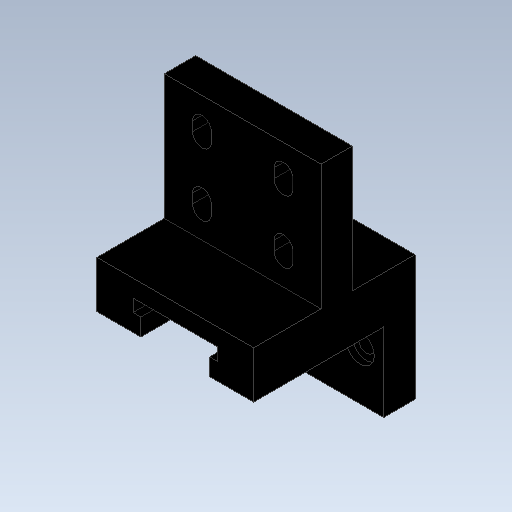
# Autodesk Inventor part: 10-03-029
Saved by Autodesk Inventor 2020 (Build 240168000, 168)
## iProperties
Created: 2019-05-27
Part Number: 10-03-029
Material: Generic
Document SubType Name: Modeling
Designer: Iulian
Density: 1 g/cm^3
Appearance: Default
Description: Suport Intinzator
Mass: 59.2019 g
Surface Area: 181.082 cm^2
Volume: 59.2019 cm^3
Author: Iulian
Subject: 037
Autodesk Inventor part; units mm, degrees
ref_plane "YZ Plane" through (0, 0, 0) normal (1, 0, 0) x (0, 1, 0)
ref_plane "XZ Plane" through (0, 0, 0) normal (0, 1, 0) x (-1, 0, 0)
sketch "Sketch1" plane through (0, 0, 0) normal (1, 0, 0) x (0, 1, 0)
  line L0 (80, 41.5) -> (25, 41.5)
  line L1 (25, 41.5) -> (25, -10)
  line L2 (25, -10) -> (80, -10)
  line L3 (80, -10) -> (80, 41.5)
  line L4 (25, 0) -> (0, 0)
  line L5 (0, 0) -> (0, -10)
  line L6 (0, -10) -> (25, -10)
  line L7 (25, -10) -> (25, 0)
  line L8 (40, 10) -> (80, 10)
  line L9 (80, 10) -> (80, -10)
  line L10 (80, -10) -> (40, -10)
  line L11 (40, -10) -> (40, 10)
  point P0 (25, -10)
  dimension "d0" = 55
  dimension "d1" = 10
  dimension "d3" = 51.5
  dimension "d135" = 25
  dimension "d144" = 20
  dimension "d145" = 40
  constraints: 24 end point, 6 parallel, 3 collinear, 3 horizontal, 3 perpendicular, 1 coincident, 1 point on line
  measures "d0" distance of L0.start L0.end
  measures "d1" distance of L4.end L5.end
  measures "d3" distance of L2.end L0.start
  measures "d135" distance between parallel lines of L1 L5
  measures "d144" distance of L10.end L8.start
  measures "d145" distance of L8.start L8.end
extrude "Extrusion1" add sketch "Sketch1" along normal blind 50 contours L3 L8 L11 L2 L1 L0 | L1 L6 L5 L4
ref_plane "Work Plane1" through (0, 25, 8.75) normal (0, 0, 1) x (1, 0, 0)
sketch "Sketch23" plane through (0, 25, 41.5) normal (0, 0, 1) x (1, 0, 0)
  line L0 (38.5, 9.5) -> (11.5, 9.5)
  line L1 (0, 0) -> (50, 0) projected
  line L2 (38.5, 9.5) -> (38.5, 5.5)
  line L3 (38.5, 5.5) -> (36, 5.5)
  line L4 (36, 5.5) -> (36, 0)
  line L5 (0, 0) -> (50, 0) projected
  line L6 (11.5, 9.5) -> (11.5, 5.5)
  line L7 (11.5, 5.5) -> (14, 5.5)
  line L8 (14, 5.5) -> (14, 0)
  point P0 (0, -25)
  point P1 (25, 9.5)
  point P2 (25, 0)
  point P3 (14, 0)
  point P4 (36, 0)
  dimension "d149" = 9.5
  dimension "d150" = 4
  dimension "d151" = 2.5
  dimension "d152" = 27
  constraints: 14 end point, 3 parallel, 3 perpendicular, 2 equal length, 2 midpoint, 2 point on line, 1 vertical, 1 vertical alignment
  measures "d149" distance between parallel lines of L0 L1
  measures "d150" distance of L0.start L2.end
  measures "d151" distance of L2.end L3.end
  measures "d152" distance of L0.start L0.end
extrude "Extrusion16" cut sketch "Sketch23" against normal up to surface (41.5 mm away)
sketch "Sketch24" plane through (50, 0, 0) normal (1, 0, 0) x (0, 0, -1)
  line L0 (-20, 45) -> (-41.5, 45)
  line L1 (-41.5, 45) -> (-41.5, 80)
  line L2 (-41.5, 80) -> (-20, 80)
  line L3 (-20, 80) -> (-20, 45)
  line L4 (-10, 40) -> (-10, 80) projected
  line L5 (10, 40) -> (-10, 40) projected
  line L6 (-41.5, 80) -> (-41.5, 25) projected
  line L7 (-10, 80) -> (-41.5, 80) projected
  point P0 (0, 0)
  dimension "d155" = 10
  dimension "d156" = 5
  constraints: 8 end point, 2 collinear, 2 parallel, 1 horizontal, 1 perpendicular
  measures "d155" distance between parallel lines of L4 L3
  measures "d156" distance between parallel lines of L0 L5
extrude "Extrusion17" cut sketch "Sketch24" against normal through all
sketch "Sketch25" plane through (0, 0, 0) normal (0, 0, 1) x (1, 0, 0)
  circle A0 centre (7.5, 15.5) radius 2.5
  circle A1 centre (42.5, 15.5) radius 2.5
  line L0 (0, 0) -> (50, 0) projected
  line L1 (50, 25) -> (50, 0) projected
  dimension "d162" = 5
  dimension "d163" = 15.5
  dimension "d164" = 7.5
  dimension "d165" = 35
  constraints: 2 centre point, 1 equal radius, 1 horizontal alignment
  measures "d162" diameter of A1
  measures "d163" distance from line of L0 A1.centre
  measures "d164" distance from line of L1 A1.centre
  measures "d165" distance of A0.centre A1.centre
hole "Hole5" at (7.5, 15.5, 0) at (42.5, 15.5, 0) direction (0, 0, -1) diameter 5 end through all counterbore diameter 9 counterbore depth 2
move faces "Move6" translate (0, -5, 0) faces at (33.3333, 45, 34.3333)
sketch "Sketch26" plane through (0, 80, 20) normal (0, 0, 1) x (1, 0, 0)
  line L0 (38, -31.5) -> (38, -28.5) construction
  line L1 (41, -31.5) -> (41, -28.5)
  line L2 (35, -28.5) -> (35, -31.5)
  arc A0 (35, -31.5) -> (41, -31.5) centre (38, -31.5) ccw
  arc A1 (41, -28.5) -> (35, -28.5) centre (38, -28.5) ccw
  line L3 (12, -31.5) -> (12, -28.5) construction
  line L4 (15, -31.5) -> (15, -28.5)
  line L5 (9, -28.5) -> (9, -31.5)
  arc A2 (9, -31.5) -> (15, -31.5) centre (12, -31.5) ccw
  arc A3 (15, -28.5) -> (9, -28.5) centre (12, -28.5) ccw
  line L6 (38, -11.5) -> (38, -8.5) construction
  line L7 (41, -11.5) -> (41, -8.5)
  line L8 (35, -8.5) -> (35, -11.5)
  arc A4 (35, -11.5) -> (41, -11.5) centre (38, -11.5) ccw
  arc A5 (41, -8.5) -> (35, -8.5) centre (38, -8.5) ccw
  line L9 (12, -11.5) -> (12, -8.5) construction
  line L10 (15, -11.5) -> (15, -8.5)
  line L11 (9, -8.5) -> (9, -11.5)
  arc A6 (9, -11.5) -> (15, -11.5) centre (12, -11.5) ccw
  arc A7 (15, -8.5) -> (9, -8.5) centre (12, -8.5) ccw
  line L12 (50, 0) -> (50, -35) projected
  line L13 (0, -35) -> (0, 0) projected
  line L14 (0, 0) -> (50, 0) projected
  line L15 (50, -40) -> (0, -40) projected
  point P0 (0, -80)
  point P1 (38, -30)
  point P2 (12, -30)
  point P3 (38, -10)
  point P4 (12, -10)
  dimension "d173" = 3
  dimension "d174" = 6
  dimension "d176" = 12
  dimension "d177" = 12
  dimension "d178" = 10
  dimension "d185" = 10
  constraints: 32 end point, 16 point on circle, 16 tangent, 8 centre point, 5 parallel, 4 midpoint, 4 point on line, 3 equal length, 3 equal radius, 2 horizontal alignment, 1 vertical, 1 vertical alignment
  measures "d173" distance of L0.start L0.end
  measures "d174" distance between parallel lines of L2 L1
  measures "d176" distance from line of point (38, -30) L12
  measures "d177" distance between parallel lines of L13 L3
  measures "d178" distance from line of L14 point (38, -10)
  measures "d185" distance from line of point (38, -30) L15
extrude "Extrusion18" cut sketch "Sketch26" against normal through all
equation "\"d177\" = d176"
equation "\"d178\" = d175"
equation "\"d175\" = 10"
body "Solid1"
